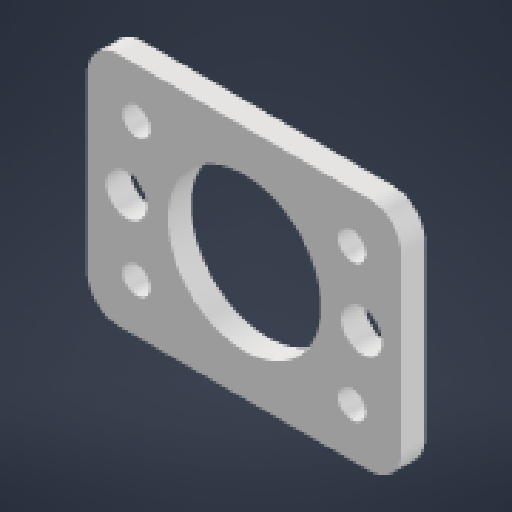
# Autodesk Inventor part: button_holder_face
Saved by Autodesk Inventor 2024.1 (Build 281209000, 209)
## iProperties
Created: 2025-01-19
Part Number: button_holder_face
Material: Generic
Document SubType Name: Modeling
Designer: Vibhu Iyer
Density: 1 g/cm^3
Appearance: Default
Author: Vibhu Iyer
Autodesk Inventor part; units mm, degrees
ref_plane "YZ Plane" through (0, 0, 0) normal (1, 0, 0) x (0, 1, 0)
ref_plane "XZ Plane" through (0, 0, 0) normal (0, 1, 0) x (-1, 0, 0)
ref_plane "XY Plane" through (0, 0, 0) normal (0, 0, 1) x (1, 0, 0)
sketch "Sketch1" plane through (0, 0, 0) normal (0, 0, 1) x (1, 0, 0)
  arc A0 (13.75, 13) -> (18, 8.75) centre (13.75, 8.75) ccw construction
  line L0 (18, -8.75) -> (18, 8.75) construction
  arc A1 (18, -8.75) -> (13.75, -13) centre (13.75, -8.75) ccw construction
  line L1 (-13.75, -13) -> (13.75, -13) construction
  arc A2 (-13.75, -13) -> (-18, -8.75) centre (-13.75, -8.75) ccw construction
  line L2 (-18, 8.75) -> (-18, -8.75) construction
  arc A3 (-18, 8.75) -> (-13.75, 13) centre (-13.75, 8.75) ccw construction
  line L3 (13.75, 13) -> (-13.75, 13) construction
  circle A4 centre (-13.75, 8.75) radius 2.25 construction
  circle A5 centre (13.75, -8.75) radius 2.25 construction
  circle A6 centre (13.75, 8.75) radius 2.25 construction
  circle A7 centre (-13.75, -8.75) radius 2.25 construction
  arc A8 (-20, -11) -> (-16, -15) centre (-16, -11) ccw projected
  line L4 (16, -15) -> (-16, -15) projected
  arc A9 (16, -15) -> (20, -11) centre (16, -11) ccw projected
  line L5 (20, 11) -> (20, -11) projected
  arc A10 (20, 11) -> (16, 15) centre (16, 11) ccw projected
  line L6 (-16, 15) -> (16, 15) projected
  arc A11 (-16, 15) -> (-20, 11) centre (-16, 11) ccw projected
  line L7 (-20, -11) -> (-20, 11) projected
  circle A12 centre (-13.75, 8.75) radius 1.75
  circle A13 centre (13.75, 8.75) radius 1.75
  circle A14 centre (13.75, -8.75) radius 1.75
  circle A15 centre (-13.75, -8.75) radius 1.75
  circle A16 centre (0, 0) radius 9.75
  circle A17 centre (-15, 0) radius 2.6
  circle A18 centre (15, 0) radius 2.6
  line L8 (-15, 0) -> (15, 0)
  dimension "d0" = 3.5
  dimension "d1" = 19.5
  dimension "d2" = 5.2
  dimension "d3" = 30
  constraints: 7 centre point, 7 coincident, 4 equal radius, 2 end point, 1 horizontal, 1 midpoint
  measures "d0" diameter of A14
  measures "d1" diameter of A16
  measures "d2" diameter of A18
  measures "d3" distance of L8.start L8.end
extrude "Extrusion1" add sketch "Sketch1" along normal blind 3
body "Solid1"
